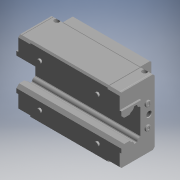
# Autodesk Inventor part: HSR35RSSB-M6F1 Slider-1-R2
Saved by Autodesk Inventor 2017.3 (Build 213256000, 256)
## iProperties
Part Number: HSR35RSSB-M6F1 Slider-1-R2
Material: Generic
Catalog Web Link: www.cadenas.de
Description: Compact Type - Heavy Load HSR-R Slider-Slider
Vendor: THK
Document SubType Name: Modeling
Designer: partserver
Manufacturer: THK
Mass: 258.114 g
Surface Area: 365.82 cm^2
Volume: 258.114 cm^3
Density: 1 g/cm^3
Appearance: PSOLRGB-192-192-192
Category: PARTsolutions
Company: THK
Title: HSR35RSSB-M6F1 Slider-1-R2
Author: Cadenas PARTsolutions
Comments: Slider
PSOL_IDENT_0: {$CADENAS_DATA\23d-libs\thk\linear_motion_systems\lm_guide\lm_guide\lm_guide_hsr\four_taped_hole_typ
PSOL_IDENT_1: e\hsr_r\hsr_r_slider.prj},241 {VTYP=3D},{NB=HSR35RSSB-M6F1 Slider-1-R2},{LINA=HSR35RSSB-M6F1 Slider-
PSOL_IDENT_2: 1-R2},{NN=Compact Type - Heavy Load HSR-R Slider},{DATE=21.06.2021 00:23:41},{GEOMDATE=11.12.2020 08
PSOL_IDENT_3: :43:00},{VERSION=},{LINEID=80},{WBVAR=SO,QZ,GPJ,TH,XY},{WBNUMERIC=XY}  {NB=HSR35RSSB-M6F1 Slider-1-R
PSOL_IDENT_4: 2},{LINA=HSR35RSSB-M6F1 Slider-1-R2},{KT=DUMMY},{REV=R2},{MN=HSR35R},{SO=SS},{QZ=},{GPJ=B-M6F},{TH=1
PSOL_IDENT_5: },{SO1='SS','SS- With end, side seals','','Without Seals','UU','UU- With end seals (on both ends)','
PSOL_IDENT_6: DD','DD- With double, side, inner seals','ZZ','ZZ- With end, side, inner seals and metal scrapers','
PSOL_IDENT_7: KK','KK- With double, side, inner seals and metal scrapers','SSHH','SSHH- With end, side, inner seal
PSOL_IDENT_8: s and LaCS','DDHH','DDHH- With double, side, inner seals and LaCS','ZZHH','ZZHH- With end, side, inn
PSOL_IDENT_9: er seals and metal scrapers and LaCS','KKHH','KKHH- With double, side, inner seals and metal scraper
PSOL_IDENT_10: s and LaCS'},{M=55.00},{W=70.00},{L=109.40},{B=50.00},{C=50.00},{S=8.00},{SL=12.000},{L1=80.40},{T=1
PSOL_IDENT_11: 1.700},{K=47.50},{N=15.00},{H3=7.500},{W1=34.000},{M1=29.000},{LX=109.4},{SH=68.00},{ST=36.717},{Z1=
PSOL_IDENT_12: 2.000},{Z2=2.000},{GPJ1=<'B-M6F','B-M6F'>,'', 'None', 'A-M6F','A-M6F','C-M6F','C-M6F', 'LF-A','LF-A'
PSOL_IDENT_13: ,'LF-B','LF-B', 'SF-A','SF-A','SF-B','SF-B'},{L4=1.5},{ND=5.000},{SE=68.000},{SE1=36.717},{SE3=2.000
PSOL_IDENT_14: },{SE4=2.000},{V=44.500},{V1=60.000},{V2=4.369},{V3=1.783},{SU=1.783},{SE2=1.783},{STT=9.000},{SEE1=
PSOL_IDENT_15: 9.000},{UP=1.783},{QZX='','No','QZ','Yes'},{LP=2},{L3=11.000},{L5=2},{S2=5.500},{L7=0.000},{XX=22.00
PSOL_IDENT_16: 0},{R=2.850},{YY=30.600},{SS=2.500},{ZZ=0.000},{GPJX=2},{X=2},{E0=5.500},{F0=12.600},{D0=5.200},{D2=
PSOL_IDENT_17: 6.200},{E1=5.500},{SD2=1.000},{XY=1},{WX=11.000},{H1=8.100},{H2=7.400},{RX=14.000},{D=6.200},{LL=5.4
PSOL_IDENT_18: 70},{TX=1.000},{NOTE=MIN}
NB: HSR35RSSB-M6F1 Slider-1-R2
NN: Compact Type - Heavy Load HSR-R Slider
NT: Slider
NBSYN: $MN.$SO.$QZ.$GPJ.$TH. Slider-$XY.-$REV.
LINA: HSR35RSSB-M6F1 Slider-1-R2
CATALOG: THK
REV: R2
MN: HSR35R
SO: SS- With end, side seals
QZ: No
GPJ: B-M6F
TH: on
M: 55
W: 70
L: 109.4
B: 50
C: 50
S: 8
SL: 12
L1: 80.4
T: 11.7
K: 47.5
N: 15
H3: 7.5
W1: 34
M1: 29
SH: 68
Z1: 2
Z2: 2
ND: 5
SE: 68
SE3: 2
SE4: 2
V: 44.5
V1: 60
V2: 4.369
V3: 1.783
SU: 1.783
SE2: 1.783
STT: 9
SEE1: 9
L3: 11
S2: 5.5
L7: 0
XX: 22
R: 2.85
YY: 30.6
SS: 2.5
ZZ: 0
E0: 5.5
F0: 12.6
D0: 5.2
D2: 6.2
E1: 5.5
SD2: 1
XY: 1
WX: 11
H1: 8.1
H2: 7.4
RX: 14
D: 6.2
LL: 5.47
TX: 1
NOTE: 0
SUPPLIER: THK
ARTICLENO: HSR35RSSB-M6F1 Slider-1-R2
BOMINFO: HSR35RSSB-M6F1 Slider-1-R2
CREATOR: CADENAS GmbH
Autodesk Inventor part; units mm, degrees
sketch "Sketch_22" plane through (0, 0, 0) normal (1, 0, 0) x (0, 1, 0)
  line L0 (46, 35) -> (35.8, 35)
  line L1 (35.8, 35) -> (35.5, 34.7)
  line L2 (35.5, 34.7) -> (3.283, 34.7)
  line L3 (3.283, 34.7) -> (1.783, 33.2)
  line L4 (1.783, 33.2) -> (1.783, -33.2)
  line L5 (1.783, -33.2) -> (3.283, -34.7)
  line L6 (3.283, -34.7) -> (35.5, -34.7)
  line L7 (35.5, -34.7) -> (35.8, -35)
  line L8 (35.8, -35) -> (46, -35)
  line L9 (46, -35) -> (47.5, -33.5)
  line L10 (47.5, -33.5) -> (47.5, -16.1)
  line L11 (47.5, -16.1) -> (46.7, -15.3)
  line L12 (46.7, -15.3) -> (46.7, -5.7)
  line L13 (46.7, -5.7) -> (47.5, -4.9)
  line L14 (47.5, -4.9) -> (47.5, 4.9)
  line L15 (47.5, 4.9) -> (46.7, 5.7)
  line L16 (46.7, 5.7) -> (46.7, 15.3)
  line L17 (46.7, 15.3) -> (47.5, 16.1)
  line L18 (47.5, 16.1) -> (47.5, 33.5)
  line L19 (47.5, 33.5) -> (46, 35)
  constraints: 40 end point
extrude "Extrusion1" add sketch "Sketch_22" along normal mid plane 80.4
sketch "Sketch2" plane through (-40.2, 47.5, 33.5) normal (0, 1, 0) x (1, 0, 0)
  point P0 (15.2, 8.5)
hole "Hole1" at (-25, 47.5, 25) direction (0, -1, 0) diameter 6.647 depth 14.4 tip angle 120 countersink diameter 8 countersink angle 90 thread size "M8x1.25" class "6H" standard "ISO Metric profile"
pattern_linear "Rectangular Pattern1" count 2 spacing 50 along (1, 0, 0) count 2 spacing 50 along (0, 0, -1) of "Hole1"
sketch "Sketch_7" plane through (-51.2, 0, 0) normal (1, 0, 0) x (0, 0, -1)
  line L0 (-34, 3.783) -> (-32, 1.783)
  line L1 (-32, 1.783) -> (32, 1.783)
  line L2 (32, 1.783) -> (34, 3.783)
  line L3 (34, 3.783) -> (34, 36.5)
  line L4 (34, 36.5) -> (32, 38.5)
  line L5 (32, 38.5) -> (-32, 38.5)
  line L6 (-32, 38.5) -> (-34, 36.5)
  line L7 (-34, 36.5) -> (-34, 3.783)
  constraints: 16 end point
extrude "Extrusion2" add sketch "Sketch_7" along normal blind 11
sketch "Sketch_2" plane through (-51.2, 0, 0) normal (1, 0, 0) x (0, 0, -1)
  line L0 (-34, 3.783) -> (-32, 1.783)
  line L1 (-32, 1.783) -> (32, 1.783)
  line L2 (32, 1.783) -> (34, 3.783)
  line L3 (34, 3.783) -> (34, 36.5)
  line L4 (34, 36.5) -> (32, 38.5)
  line L5 (32, 38.5) -> (-32, 38.5)
  line L6 (-32, 38.5) -> (-34, 36.5)
  line L7 (-34, 36.5) -> (-34, 3.783)
  constraints: 16 end point
extrude "Extrusion3" add sketch "Sketch_2" against normal blind 3.5
sketch "Sketch_8" plane through (51.2, 0, 0) normal (1, 0, 0) x (0, 0, -1)
  line L0 (-34, 3.783) -> (-32, 1.783)
  line L1 (-32, 1.783) -> (32, 1.783)
  line L2 (32, 1.783) -> (34, 3.783)
  line L3 (34, 3.783) -> (34, 36.5)
  line L4 (34, 36.5) -> (32, 38.5)
  line L5 (32, 38.5) -> (-32, 38.5)
  line L6 (-32, 38.5) -> (-34, 36.5)
  line L7 (-34, 36.5) -> (-34, 3.783)
  constraints: 16 end point
extrude "Extrusion4" add sketch "Sketch_8" against normal blind 11
sketch "Sketch_42" plane through (51.2, 0, 0) normal (1, 0, 0) x (0, 0, -1)
  line L0 (-34, 3.783) -> (-32, 1.783)
  line L1 (-32, 1.783) -> (32, 1.783)
  line L2 (32, 1.783) -> (34, 3.783)
  line L3 (34, 3.783) -> (34, 36.5)
  line L4 (34, 36.5) -> (32, 38.5)
  line L5 (32, 38.5) -> (-32, 38.5)
  line L6 (-32, 38.5) -> (-34, 36.5)
  line L7 (-34, 36.5) -> (-34, 3.783)
  constraints: 16 end point
extrude "Extrusion5" add sketch "Sketch_42" along normal blind 3.5
sketch "Sketch_106" plane through (40.2, 0, 0) normal (1, 0, 0) x (0, 0, -1)
  line L0 (-9.8715, 39.4) -> (-9.8715, 37.9)
  line L1 (-9.8715, 37.9) -> (9.8715, 37.9)
  line L2 (9.8715, 37.9) -> (9.8715, 39.4)
  arc A0 (5.5, 40.1) -> (9.8715, 39.4) centre (9.8715, 53.4) ccw
  line L3 (5.5, 40.1) -> (-5.5, 40.1)
  arc A1 (-9.8715, 39.4) -> (-5.5, 40.1) centre (-9.8715, 53.4) ccw
  constraints: 8 end point, 4 point on circle, 2 centre point
extrude "Extrusion6" add sketch "Sketch_106" along normal blind 10.5
sketch "Sketch_107" plane through (-40.2, 0, 0) normal (1, 0, 0) x (0, 0, -1)
  line L0 (-9.8715, 39.4) -> (-9.8715, 37.9)
  line L1 (-9.8715, 37.9) -> (9.8715, 37.9)
  line L2 (9.8715, 37.9) -> (9.8715, 39.4)
  arc A0 (5.5, 40.1) -> (9.8715, 39.4) centre (9.8715, 53.4) ccw
  line L3 (5.5, 40.1) -> (-5.5, 40.1)
  arc A1 (-9.8715, 39.4) -> (-5.5, 40.1) centre (-9.8715, 53.4) ccw
  constraints: 8 end point, 4 point on circle, 2 centre point
extrude "Extrusion7" add sketch "Sketch_107" against normal blind 10.5
sketch "Sketch9" plane through (-50.7, 40.1, -5.5) normal (0, 1, 0) x (1, 0, 0)
  point P0 (5.03, -5.5)
hole "Hole2" at (-45.67, 40.1, 0) direction (0, -1, 0) diameter 6.2 depth 1
sketch "Sketch10" plane through (40.2, 40.1, 5.5) normal (0, 1, 0) x (1, 0, 0)
  point P0 (5.47, 5.5)
hole "Hole3" at (45.67, 40.1, 0) direction (0, -1, 0) diameter 6.2 depth 1
sketch "Sketch_1" plane through (54.7, 0, 0) normal (1, 0, 0) x (0, 0, -1)
  line L0 (-34, 47.5) -> (-34, 0)
  line L1 (-34, 0) -> (34, 0)
  line L2 (34, 0) -> (34, 47.5)
  line L3 (34, 47.5) -> (-34, 47.5)
  constraints: 8 end point
extrude "Extrusion8" cut sketch "Sketch_1" against normal blind 2
sketch "Sketch_6" plane through (-54.7, 0, 0) normal (1, 0, 0) x (0, 0, -1)
  line L0 (-34, 47.5) -> (-34, 0)
  line L1 (-34, 0) -> (34, 0)
  line L2 (34, 0) -> (34, 47.5)
  line L3 (34, 47.5) -> (-34, 47.5)
  constraints: 8 end point
extrude "Extrusion9" cut sketch "Sketch_6" along normal blind 2
sketch "Sketch_20" plane through (-52.7, 0, 0) normal (1, 0, 0) x (0, 0, -1)
  line L0 (-19, 1.783) -> (19, 1.783)
  line L1 (19, 1.783) -> (19, 22.5)
  line L2 (19, 22.5) -> (18, 23.5)
  line L3 (18, 23.5) -> (-18, 23.5)
  line L4 (-18, 23.5) -> (-19, 22.5)
  line L5 (-19, 22.5) -> (-19, 1.783)
  constraints: 12 end point
extrude "Extrusion10" add sketch "Sketch_20" against normal blind 2
sketch "Sketch_21" plane through (52.7, 0, 0) normal (1, 0, 0) x (0, 0, -1)
  line L0 (-19, 1.783) -> (19, 1.783)
  line L1 (19, 1.783) -> (19, 22.5)
  line L2 (19, 22.5) -> (18, 23.5)
  line L3 (18, 23.5) -> (-18, 23.5)
  line L4 (-18, 23.5) -> (-19, 22.5)
  line L5 (-19, 22.5) -> (-19, 1.783)
  constraints: 12 end point
extrude "Extrusion11" add sketch "Sketch_21" along normal blind 2
sketch "Sketch_65" plane through (0, 0, 0) normal (1, 0, 0) x (0, 1, 0)
  line L0 (-0.4998, 17) -> (-0.4998, -17)
  line L1 (-0.4998, -17) -> (4.6999, -11.8003)
  line L2 (4.6999, -11.8003) -> (10.1796, -11.8003)
  line L3 (10.1796, -11.8003) -> (12.0174, -13.6381)
  arc A0 (14.8609, -16.4816) -> (12.0174, -13.6381) centre (11.5889, -16.9102) ccw
  line L4 (14.8609, -16.4816) -> (15.3793, -17)
  line L5 (15.3793, -17) -> (17.6102, -17)
  line L6 (17.6102, -17) -> (18.1415, -16.4686)
  arc A1 (20.9703, -13.6398) -> (18.1415, -16.4686) centre (21.4119, -16.9102) ccw
  line L7 (20.9703, -13.6398) -> (21.5, -13.1102)
  line L8 (21.5, -13.1102) -> (21.5, 13.1102)
  line L9 (21.5, 13.1102) -> (20.9703, 13.6398)
  arc A2 (18.1415, 16.4686) -> (20.9703, 13.6398) centre (21.4119, 16.9102) ccw
  line L10 (18.1415, 16.4686) -> (17.6102, 17)
  line L11 (17.6102, 17) -> (15.3793, 17)
  line L12 (15.3793, 17) -> (14.8609, 16.4816)
  arc A3 (12.0174, 13.6381) -> (14.8609, 16.4816) centre (11.5889, 16.9102) ccw
  line L13 (12.0174, 13.6381) -> (10.1796, 11.8003)
  line L14 (10.1796, 11.8003) -> (4.6999, 11.8003)
  line L15 (4.6999, 11.8003) -> (-0.4998, 17)
  constraints: 32 end point, 8 point on circle, 4 centre point
extrude "Extrusion12" cut sketch "Sketch_65" along normal mid plane 109.4
sketch "Sketch_4" plane through (0, 0, -11) normal (0, 0, 1) x (1, 0, 0)
  line L0 (54.2, 30.6) -> (52.7, 30.6)
  line L1 (52.7, 30.6) -> (52.7, 33.45)
  line L2 (52.7, 33.45) -> (53.825, 33.45)
  arc A0 (54.2, 33.075) -> (53.825, 33.45) centre (53.825, 33.075) ccw
  line L3 (54.2, 33.075) -> (54.2, 30.6)
  line L4 (54.2, 30.6) -> (52.7, 30.6)
  constraints: 10 end point, 2 point on circle, 1 centre point
revolve "Revolution1" add sketch "Sketch_4" angle 360 about axis through (54.2, 30.6, -11) along (1, 0, 0)
sketch "Sketch_14" plane through (0, 0, -11) normal (0, 0, 1) x (1, 0, 0)
  line L0 (-52.7, 30.6) -> (-54.2, 30.6)
  line L1 (-54.2, 30.6) -> (-54.2, 33.075)
  arc A0 (-53.825, 33.45) -> (-54.2, 33.075) centre (-53.825, 33.075) ccw
  line L2 (-53.825, 33.45) -> (-52.7, 33.45)
  line L3 (-52.7, 33.45) -> (-52.7, 30.6)
  line L4 (-52.7, 30.6) -> (-54.2, 30.6)
  constraints: 10 end point, 2 point on circle, 1 centre point
revolve "Revolution2" add sketch "Sketch_14" angle 360 about axis through (-52.7, 30.6, -11) along (1, 0, 0)
sketch "Sketch_15" plane through (0, 0, 11) normal (0, 0, 1) x (1, 0, 0)
  line L0 (54.2, 30.6) -> (52.7, 30.6)
  line L1 (52.7, 30.6) -> (52.7, 33.45)
  line L2 (52.7, 33.45) -> (53.825, 33.45)
  arc A0 (54.2, 33.075) -> (53.825, 33.45) centre (53.825, 33.075) ccw
  line L3 (54.2, 33.075) -> (54.2, 30.6)
  line L4 (54.2, 30.6) -> (52.7, 30.6)
  constraints: 10 end point, 2 point on circle, 1 centre point
revolve "Revolution3" add sketch "Sketch_15" angle 360 about axis through (54.2, 30.6, 11) along (1, 0, 0)
sketch "Sketch_16" plane through (0, 0, 11) normal (0, 0, 1) x (1, 0, 0)
  line L0 (-52.7, 30.6) -> (-54.2, 30.6)
  line L1 (-54.2, 30.6) -> (-54.2, 33.075)
  arc A0 (-53.825, 33.45) -> (-54.2, 33.075) centre (-53.825, 33.075) ccw
  line L2 (-53.825, 33.45) -> (-52.7, 33.45)
  line L3 (-52.7, 33.45) -> (-52.7, 30.6)
  line L4 (-52.7, 30.6) -> (-54.2, 30.6)
  constraints: 10 end point, 2 point on circle, 1 centre point
revolve "Revolution4" add sketch "Sketch_16" angle 360 about axis through (-52.7, 30.6, 11) along (1, 0, 0)
sketch "Sketch_24" plane through (54.2, 0, 0) normal (1, 0, 0) x (0, 0, -1)
  line L0 (9.75, 29.8783) -> (11, 29.1566)
  line L1 (11, 29.1566) -> (12.25, 29.8783)
  line L2 (12.25, 29.8783) -> (12.25, 31.3217)
  line L3 (12.25, 31.3217) -> (11, 32.0434)
  line L4 (11, 32.0434) -> (9.75, 31.3217)
  line L5 (9.75, 31.3217) -> (9.75, 29.8783)
  constraints: 12 end point
extrude "Extrusion13" cut sketch "Sketch_24" against normal blind 0.75
sketch "Sketch_25" plane through (54.2, 0, 0) normal (1, 0, 0) x (0, 0, -1)
  line L0 (-12.25, 29.8783) -> (-11, 29.1566)
  line L1 (-11, 29.1566) -> (-9.75, 29.8783)
  line L2 (-9.75, 29.8783) -> (-9.75, 31.3217)
  line L3 (-9.75, 31.3217) -> (-11, 32.0434)
  line L4 (-11, 32.0434) -> (-12.25, 31.3217)
  line L5 (-12.25, 31.3217) -> (-12.25, 29.8783)
  constraints: 12 end point
extrude "Extrusion14" cut sketch "Sketch_25" against normal blind 0.75
sketch "Sketch_26" plane through (-54.2, 0, 0) normal (1, 0, 0) x (0, 0, -1)
  line L0 (9.75, 29.8783) -> (11, 29.1566)
  line L1 (11, 29.1566) -> (12.25, 29.8783)
  line L2 (12.25, 29.8783) -> (12.25, 31.3217)
  line L3 (12.25, 31.3217) -> (11, 32.0434)
  line L4 (11, 32.0434) -> (9.75, 31.3217)
  line L5 (9.75, 31.3217) -> (9.75, 29.8783)
  constraints: 12 end point
extrude "Extrusion15" cut sketch "Sketch_26" along normal blind 0.75
sketch "Sketch_27" plane through (-54.2, 0, 0) normal (1, 0, 0) x (0, 0, -1)
  line L0 (-12.25, 29.8783) -> (-11, 29.1566)
  line L1 (-11, 29.1566) -> (-9.75, 29.8783)
  line L2 (-9.75, 29.8783) -> (-9.75, 31.3217)
  line L3 (-9.75, 31.3217) -> (-11, 32.0434)
  line L4 (-11, 32.0434) -> (-12.25, 31.3217)
  line L5 (-12.25, 31.3217) -> (-12.25, 29.8783)
  constraints: 12 end point
extrude "Extrusion16" cut sketch "Sketch_27" along normal blind 0.75
sketch "Sketch_12" plane through (0, 0, 0) normal (0, 0, 1) x (1, 0, 0)
  line L0 (-51.2, 38) -> (-50.7, 38.5)
  line L1 (-50.7, 38.5) -> (-51.2, 38.5)
  line L2 (-51.2, 38.5) -> (-51.2, 38)
  constraints: 6 end point
extrude "Extrusion17" cut sketch "Sketch_12" along normal mid plane 68
sketch "Sketch_13" plane through (0, 0, 0) normal (0, 0, 1) x (1, 0, 0)
  line L0 (50.7, 38.5) -> (51.2, 38)
  line L1 (51.2, 38) -> (51.2, 38.5)
  line L2 (51.2, 38.5) -> (50.7, 38.5)
  constraints: 6 end point
extrude "Extrusion18" cut sketch "Sketch_13" along normal mid plane 68
sketch "Sketch_45" plane through (0, 0, 0) normal (0, 1, 0) x (-1, 0, 0)
  line L0 (-50.7, -34) -> (-51.2, -33.5)
  line L1 (-51.2, -33.5) -> (-51.2, -34)
  line L2 (-51.2, -34) -> (-50.7, -34)
  constraints: 6 end point
extrude "Extrusion19" cut sketch "Sketch_45" along normal blind 47.5
sketch "Sketch_46" plane through (0, 0, 0) normal (0, 1, 0) x (-1, 0, 0)
  line L0 (51.2, -33.5) -> (50.7, -34)
  line L1 (50.7, -34) -> (51.2, -34)
  line L2 (51.2, -34) -> (51.2, -33.5)
  constraints: 6 end point
extrude "Extrusion20" cut sketch "Sketch_46" along normal blind 47.5
sketch "Sketch_47" plane through (0, 0, 0) normal (0, 1, 0) x (-1, 0, 0)
  line L0 (-50.7, 34) -> (-51.2, 34)
  line L1 (-51.2, 34) -> (-51.2, 33.5)
  line L2 (-51.2, 33.5) -> (-50.7, 34)
  constraints: 6 end point
extrude "Extrusion21" cut sketch "Sketch_47" along normal blind 47.5
sketch "Sketch_48" plane through (0, 0, 0) normal (0, 1, 0) x (-1, 0, 0)
  line L0 (51.2, 33.5) -> (51.2, 34)
  line L1 (51.2, 34) -> (50.7, 34)
  line L2 (50.7, 34) -> (51.2, 33.5)
  constraints: 6 end point
extrude "Extrusion22" cut sketch "Sketch_48" along normal blind 47.5
sketch "Sketch30" plane through (52.7, 0, 0) normal (1, 0, 0) x (0, 0, -1)
  point P0 (0, 32.5)
hole "Hole4" at (52.7, 32.5, 0) direction (-1, 0, 0) diameter 4.917 depth 6 tip angle 120 countersink diameter 6 countersink angle 90 thread size "M6x1" class "6H" standard "ISO Metric profile"
sketch "Sketch31" plane through (-52.7, 0, 0) normal (-1, 0, 0) x (0, 0, 1)
  point P0 (0, 32.5)
hole "Hole5" at (-52.7, 32.5, 0) direction (1, 0, 0) diameter 4.917 depth 6 tip angle 120 countersink diameter 6 countersink angle 90 thread size "M6x1" class "6H" standard "ISO Metric profile"
sketch "Sketch_34" plane through (0, 0, -22.25) normal (0, 0, 1) x (1, 0, 0)
  line L0 (-30, 4.369) -> (-30, 0)
  line L1 (-30, 0) -> (-31.7476, 0)
  arc A0 (-32.1845, 0.4369) -> (-31.7476, 0) centre (-31.7476, 0.4369) ccw
  line L2 (-32.1845, 0.4369) -> (-32.1845, 4.369)
  line L3 (-32.1845, 4.369) -> (-30, 4.369)
  line L4 (-30, 4.369) -> (-30, 0)
  constraints: 10 end point, 2 point on circle, 1 centre point
revolve "Revolution5" add sketch "Sketch_34" angle 360 about axis through (-30, 4.369, -22.25) along (0, 1, 0)
sketch "Sketch_35" plane through (0, 0, -22.25) normal (0, 0, 1) x (1, 0, 0)
  line L0 (30, 4.369) -> (30, 0)
  line L1 (30, 0) -> (28.2524, 0)
  arc A0 (27.8155, 0.4369) -> (28.2524, 0) centre (28.2524, 0.4369) ccw
  line L2 (27.8155, 0.4369) -> (27.8155, 4.369)
  line L3 (27.8155, 4.369) -> (30, 4.369)
  line L4 (30, 4.369) -> (30, 0)
  constraints: 10 end point, 2 point on circle, 1 centre point
revolve "Revolution6" add sketch "Sketch_35" angle 360 about axis through (30, 4.369, -22.25) along (0, 1, 0)
sketch "Sketch_37" plane through (0, 0, 22.25) normal (0, 0, 1) x (1, 0, 0)
  line L0 (-30, 4.369) -> (-30, 0)
  line L1 (-30, 0) -> (-31.7476, 0)
  arc A0 (-32.1845, 0.4369) -> (-31.7476, 0) centre (-31.7476, 0.4369) ccw
  line L2 (-32.1845, 0.4369) -> (-32.1845, 4.369)
  line L3 (-32.1845, 4.369) -> (-30, 4.369)
  line L4 (-30, 4.369) -> (-30, 0)
  constraints: 10 end point, 2 point on circle, 1 centre point
revolve "Revolution7" add sketch "Sketch_37" angle 360 about axis through (-30, 4.369, 22.25) along (0, 1, 0)
sketch "Sketch_38" plane through (0, 0, 22.25) normal (0, 0, 1) x (1, 0, 0)
  line L0 (30, 4.369) -> (30, 0)
  line L1 (30, 0) -> (28.2524, 0)
  arc A0 (27.8155, 0.4369) -> (28.2524, 0) centre (28.2524, 0.4369) ccw
  line L2 (27.8155, 0.4369) -> (27.8155, 4.369)
  line L3 (27.8155, 4.369) -> (30, 4.369)
  line L4 (30, 4.369) -> (30, 0)
  constraints: 10 end point, 2 point on circle, 1 centre point
revolve "Revolution8" add sketch "Sketch_38" angle 360 about axis through (30, 4.369, 22.25) along (0, 1, 0)
sketch "Sketch_94" plane through (45.7, 0, 0) normal (1, 0, 0) x (0, 0, -1)
  line L0 (-28.8, 34.9) -> (-34, 34.9)
  line L1 (-34, 34.9) -> (-34, 37.5)
  line L2 (-34, 37.5) -> (-28.8, 37.5)
  line L3 (-28.8, 37.5) -> (-28.8, 34.9)
  line L4 (-28.8, 34.9) -> (-34, 34.9)
  constraints: 10 end point
revolve "Revolution9" cut sketch "Sketch_94" angle 360 about axis through (45.7, 34.9, 28.8) along (0, 0, -1)
sketch "Sketch37" plane through (40.2, 3.783, -34) normal (0, 0, -1) x (-1, 0, 0)
  point P0 (-5.5, 31.117)
hole "Hole6" at (45.7, 34.9, -34) direction (0, 0, 1) diameter 5.2 depth 5.2
sketch "Sketch_96" plane through (-45.7, 0, 0) normal (1, 0, 0) x (0, 0, -1)
  line L0 (-28.8, 34.9) -> (-34, 34.9)
  line L1 (-34, 34.9) -> (-34, 37.5)
  line L2 (-34, 37.5) -> (-28.8, 37.5)
  line L3 (-28.8, 37.5) -> (-28.8, 34.9)
  line L4 (-28.8, 34.9) -> (-34, 34.9)
  constraints: 10 end point
revolve "Revolution10" cut sketch "Sketch_96" angle 360 about axis through (-45.7, 34.9, 28.8) along (0, 0, -1)
sketch "Sketch39" plane through (-40.2, 3.783, -34) normal (0, 0, -1) x (-1, 0, 0)
  point P0 (5.5, 31.117)
hole "Hole7" at (-45.7, 34.9, -34) direction (0, 0, 1) diameter 5.2 depth 5.2
ref_plane "4TRACK_XY" through (0, 0, 0) normal (1, 0, 0) x (0, 0, -1)
ref_plane "4TRACK_YZ" through (0, 0, 0) normal (0, 0, -1) x (0, 1, 0)
ref_plane "4TRACK_ZX" through (0, 0, 0) normal (0, 1, 0) x (1, 0, 0)
ref_plane "niple_XY" through (-52.7, 32.5, 0) normal (1, 0, 0) x (0, 0, -1)
ref_plane "niple_YZ" through (-52.7, 32.5, 0) normal (0, 0, -1) x (0, 1, 0)
ref_plane "niple_ZX" through (-52.7, 32.5, 0) normal (0, 1, 0) x (1, 0, 0)
ref_plane "niple2_XY" through (52.7, 32.5, 0) normal (1, 0, 0) x (0, 0, -1)
ref_plane "niple2_YZ" through (52.7, 32.5, 0) normal (0, 0, -1) x (0, 1, 0)
ref_plane "niple2_ZX" through (52.7, 32.5, 0) normal (0, 1, 0) x (1, 0, 0)
body "Solid1"
